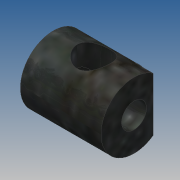
# Autodesk Inventor part: Schließbahn_ra8846s
Saved by Autodesk Inventor 2021 (Build 250183000, 183)
## iProperties
Created: 2020-12-19
Part Number: Schließbahn_ra8846s
Material: Stahl
Document SubType Name: Modeling
Designer: Ricardo
Density: 7.85 g/cm^3
Appearance: Platte
Project: Motor
Mass: 3.75138 g
Surface Area: 5.83468 cm^2
Volume: 0.477883 cm^3
Author: Sander
Revision Number: Rev00
Autodesk Inventor part; units mm, degrees
ref_plane "YZ-Ebene" through (0, 0, 0) normal (1, 0, 0) x (0, 1, 0)
ref_plane "XZ-Ebene" through (0, 0, 0) normal (0, 1, 0) x (-1, 0, 0)
sketch "Skizze1" plane through (0, 0, 0) normal (0, 0, 1) x (1, 0, 0)
  line L0 (-14.4, 0) -> (2.4, 0) projected
  line L1 (0, -0.9) -> (0, 5.4) projected
  line L2 (-12, 1.7) -> (-12, 2)
  line L3 (-12, 2) -> (-11, 2)
  line L4 (-11, 2) -> (-11, 4.5)
  line L5 (-11, 4.5) -> (0, 4.5)
  line L6 (-12, 1.7) -> (0, 1.7)
  line L7 (0, 4.5) -> (0, 1.7)
  point P0 (0, 0)
  dimension "d1" = 3.4
  dimension "d2" = 4
  dimension "d3" = 11
  dimension "d4" = 12
  dimension "d5" = 9
  constraints: 12 end point, 5 perpendicular, 2 point on line, 1 vertical
  measures "d1" diameter of L2.start L0
  measures "d2" diameter of L2.end L0
  measures "d3" distance of L4.end L5.end
  measures "d4" horizontal distance of L5.end L2.end
  measures "d5" diameter of L5.end L0
revolve "Umdrehung1" add sketch "Skizze1" angle 360 about axis through (-10, 0, 0) along (1, 0, 0)
ref_plane "Arbeitsebene1" through (-5.5, 0, 4.5) normal (0, 0, 1) x (1, 0, 0)
sketch "Skizze2" plane through (-5.5, 0, 4.5) normal (0, 0, 1) x (1, 0, 0)
  line L0 (-5.5, 4.5) -> (5.5, 4.5) projected
  line L1 (5.5, -4.5) -> (5.5, 4.5) projected
  line L2 (3, 4.5) -> (5.5, 4.5)
  line L3 (5.5, 4.5) -> (5.5, 2.6)
  line L4 (5.5, 2.6) -> (3, 2.6)
  line L5 (3, 2.6) -> (3, 4.5)
  point P0 (5.5, 0)
  dimension "d9" = 1.9
  dimension "d10" = 2.5
  constraints: 8 end point, 2 parallel, 2 point on line, 1 horizontal, 1 perpendicular
  measures "d9" distance of L4.end L2.start
  measures "d10" distance of L3.end L4.end
extrude "Extrusion1" cut sketch "Skizze2" against normal through all
ref_plane "Arbeitsebene2" through (-5.5, 0, 4.5) normal (0, 0, 1) x (1, 0, 0)
sketch "Skizze3" plane through (-5.5, 0, 4.5) normal (0, 0, 1) x (1, 0, 0)
  line L0 (-8.9, 0) -> (7.9, 0) projected
  line L1 (-5.5, -4.5) -> (-5.5, 4.5) projected
  line L2 (5.5, -4.5) -> (5.5, 2.6) projected
  circle A0 centre (0, 0) radius 2.25
  point P0 (5.5, 0)
  dimension "d13" = 4.5
  dimension "d14" = 5.5
  constraints: 1 centre point, 1 point on line, 1 other
  measures "d13" diameter of A0
  measures "d14" distance from line of L2 A0.centre
extrude "Extrusion2" cut sketch "Skizze3" against normal through all
